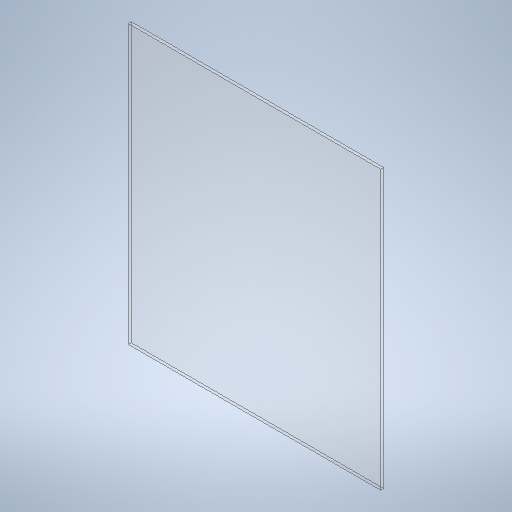
# Autodesk Inventor part: basement door right
Saved by Autodesk Inventor 2025 (Build 290162010, 162A)
## iProperties
Created: 2024-06-17
Part Number: basement door right
Material: Polycarbonate, Clear
Document SubType Name: Modeling
Designer: Alan Thomas
Mass: 4869.24 g
Surface Area: 10372.4 cm^2
Volume: 4057.7 cm^3
Density: 1.2 g/cm^3
Appearance: Polycarbonate - Clear
Author: Alan Thomas
Autodesk Inventor part; units mm, degrees
ref_plane "YZ Plane" through (0, 0, 0) normal (1, 0, 0) x (0, 1, 0)
ref_plane "XZ Plane" through (0, 0, 0) normal (0, 1, 0) x (-1, 0, 0)
ref_plane "XY Plane" through (0, 0, 0) normal (0, 0, 1) x (1, 0, 0)
sketch "Sketch1" plane through (0, 0, 0) normal (0, 0, 1) x (1, 0, 0)
  line L0 (0, 0) -> (679, 0)
  line L1 (679, 0) -> (679, 747)
  line L2 (679, 747) -> (0, 747)
  line L3 (0, 747) -> (0, 0)
  dimension "d0" = 679
  dimension "d1" = 747
  constraints: 8 end point, 2 parallel, 1 horizontal, 1 perpendicular
  measures "d0" distance of L2.end L1.end
  measures "d1" distance of L1.end L0.end
extrude "Extrusion1" add sketch "Sketch1" along normal blind 8
body "Solid1"
